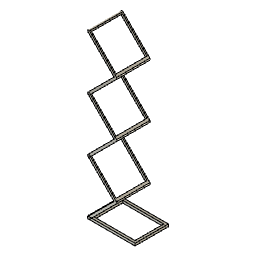
rgiro_haitian_magazine_rack (Autodesk Fusion 360 design; units mm, degrees)
Autodesk Fusion 360 part; units mm, degrees
sketch "Sketch1" plane through (0, 0, 0) normal (0, 0, 1) x (1, 0, 0)
  line L0 (-202.5, -142.5) -> (202.5, -142.5)
  line L1 (202.5, -142.5) -> (202.5, 142.5)
  line L2 (202.5, 142.5) -> (-202.5, 142.5)
  line L3 (-202.5, 142.5) -> (-202.5, -142.5)
  line L4 (-202.5, -142.5) -> (202.5, 142.5) construction
  line L5 (202.5, -142.5) -> (-202.5, 142.5) construction
  dimension "d1" = 405
  dimension "d2" = 285
  constraint perpendicular L0 L1
  constraint parallel L0 L2
  constraint parallel L1 L3
  constraint horizontal L0
  constraint coincident L4 origin
  constraint coincident L5 origin
  measures "d1" distance of L0.start L0.end
  measures "d2" distance of L0.start L2.end
extrude "Extrude1" add sketch "Sketch1" along normal blind 20 makes body 1
sketch "Sketch2" plane through (0, 0, 0) normal (0, 1, 0) x (1, 0, 0)
  line L0 (44.5711, -232.9289) -> (-185.4289, -2.9289)
  arc A0 (-185.4289, -2.9289) -> (-199.5711, -17.0711) centre (-192.5, -10) ccw
  line L1 (-199.5711, -17.0711) -> (30.4289, -247.0711)
  arc A1 (30.4289, -247.0711) -> (44.5711, -232.9289) centre (37.5, -240) ccw
  line L2 (37.5, -240) -> (-192.5, -10) construction
  line L3 (202.5, 0) -> (-202.5, 0)
  line L4 (-202.5, 0) -> (-202.5, -20)
  line L5 (30.4289, -232.9289) -> (-199.5711, -462.9289)
  arc A2 (-199.5711, -462.9289) -> (-185.4289, -477.0711) centre (-192.5, -470) ccw
  line L6 (-185.4289, -477.0711) -> (44.5711, -247.0711)
  arc A3 (44.5711, -247.0711) -> (30.4289, -232.9289) centre (37.5, -240) ccw
  line L7 (37.5, -240) -> (-192.5, -470) construction
  point P0 (-192.5, -10)
  point P1 (37.5, -240)
  dimension "d5" = 20
  dimension "d7" = 10
  dimension "d8" = 10
  dimension "d9" = 230
  dimension "d10" = 230
  dimension "d11" = 10
  dimension "d12" = 230
  dimension "d13" = 230
  constraint tangent L0 A0
  constraint tangent A0 L1
  constraint parallel L0 L1
  constraint tangent L1 A1
  constraint tangent L0 A1
  constraint coincident P1 A1.centre
  constraint coincident P0 A0.centre
  constraint tangent L5 A2
  constraint tangent A2 L6
  constraint parallel L5 L6
  constraint tangent L6 A3
  constraint tangent L5 A3
  measures "d5" distance of L0 L1
  measures "d7" distance of P0 L3
  measures "d8" distance of P0 L4
  measures "d9" horizontal distance of P0 P1
  measures "d10" vertical distance of P0 P1
  measures "d11" radius of A2
  measures "d12" horizontal distance of P1 A2.centre
  measures "d13" vertical distance of P1 A2.centre
extrude "Extrude2" add sketch "Sketch2" along normal up to surface (142.5 mm away) and the other way up to surface (142.5 mm away) separate body contours L0 A0 L1 L5 A3 | L1 A1 L5 A3 | L1 A1 L5 A2 L6 makes body 2
sketch "Sketch3" plane through (-108.3211, 0, 108.3211) normal (-0.707107, 0, 0.707107) x (0, -1, 0)
  line L0 (-142.5, 186.2221) -> (-142.5, -129.047)
  line L1 (-142.5, -129.047) -> (142.5, -129.047)
  line L2 (142.5, -129.047) -> (142.5, 186.2221)
  line L3 (142.5, 186.2221) -> (-142.5, 186.2221)
  line L4 (-132.5, -119.047) -> (132.5, -119.047)
  line L5 (132.5, -119.047) -> (132.5, 176.2221)
  line L6 (132.5, 176.2221) -> (-132.5, 176.2221)
  line L7 (-132.5, 176.2221) -> (-132.5, -119.047)
  dimension "d18" = -10
extrude "Extrude3" cut sketch "Sketch3" against normal up to surface (20 mm away) contours L4 L5 L6 L7 bodies 1 2
sketch "Sketch4" plane through (131.6789, 0, 131.6789) normal (-0.707107, 0, -0.707107) x (0, -1, 0)
  line L0 (-142.5, 468.4582) -> (-142.5, 153.1891)
  line L1 (-142.5, 153.1891) -> (142.5, 153.1891)
  line L2 (142.5, 153.1891) -> (142.5, 468.4582)
  line L3 (142.5, 468.4582) -> (-142.5, 468.4582)
  line L4 (-132.5, 163.1891) -> (132.5, 163.1891)
  line L5 (132.5, 163.1891) -> (132.5, 458.4582)
  line L6 (132.5, 458.4582) -> (-132.5, 458.4582)
  line L7 (-132.5, 458.4582) -> (-132.5, 163.1891)
  dimension "d21" = -10
extrude "Extrude4" cut sketch "Sketch4" against normal up to surface (20 mm away) contours L4 L5 L6 L7 bodies 2
pattern_linear "R-Pattern1" count 3 spacing 460 along (0, 0, 1) of bodies 2 makes body 3 at (39.857, -44.1667, 688.2149) makes body 4 at (39.857, 44.1667, 1171.7851)
sketch "Sketch5" plane through (0, 0, 20) normal (0, 0, 1) x (-1, 0, 0)
  line L0 (188.3579, -132.5) -> (168.3579, -132.5)
  line L1 (168.3579, -132.5) -> (168.3579, 132.5)
  line L2 (168.3579, 132.5) -> (188.3579, 132.5)
  line L3 (188.3579, 132.5) -> (188.3579, -132.5)
  line L4 (202.5, -142.5) -> (202.5, 142.5)
  line L5 (202.5, 142.5) -> (-202.5, 142.5)
  line L6 (-202.5, 142.5) -> (-202.5, -142.5)
  line L7 (-202.5, -142.5) -> (202.5, -142.5)
  line L8 (182.5, 122.5) -> (-182.5, 122.5)
  line L9 (-182.5, 122.5) -> (-182.5, -122.5)
  line L10 (-182.5, -122.5) -> (182.5, -122.5)
  line L11 (182.5, -122.5) -> (182.5, 122.5)
  dimension "d28" = -20
extrude "Extrude5" cut sketch "Sketch5" against normal up to surface (20 mm away) contours L1 L8 L9 L10 bodies 1
